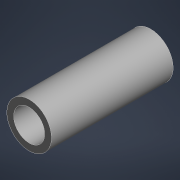
# Autodesk Inventor part: P023-Cage_arbre
Saved by Autodesk Inventor 2021.3 (Build 253353000, 353)
## iProperties
Created: 2022-06-06
Part Number: P023-Cage_arbre
Material: Générique
Document SubType Name: Modeling
Designer: Rémi Heredero
Density: 1 g/cm^3
Appearance: Par défaut
Author: Rémi Heredero
Autodesk Inventor part; units mm, degrees
ref_plane "YZ Plane" through (0, 0, 0) normal (1, 0, 0) x (0, 1, 0)
ref_plane "XZ Plane" through (0, 0, 0) normal (0, 1, 0) x (-1, 0, 0)
ref_plane "XY Plane" through (0, 0, 0) normal (0, 0, 1) x (1, 0, 0)
sketch "Sketch3" plane through (0, 0, 0) normal (1, 0, 0) x (0, 1, 0)
  line L0 (-45, 16.5) -> (-45, 11.5)
  line L1 (-45, 11.5) -> (-25, 11.5)
  line L2 (-25, 11.5) -> (-25, 11)
  line L3 (-25, 11) -> (25, 11)
  line L4 (25, 11) -> (25, 11.5)
  line L5 (25, 11.5) -> (45, 11.5)
  line L6 (45, 11.5) -> (45, 16.5)
  line L7 (45, 16.5) -> (-45, 16.5)
  line L8 (-63, 0) -> (63, 0) projected
  point P0 (0, 0)
  point P1 (0, 11)
  dimension "d0" = 5
  dimension "d1" = 20
  dimension "d2" = 50
  dimension "d6" = 23
  dimension "d7" = 22
  constraints: 16 end point, 6 perpendicular, 2 point on line, 1 collinear, 1 midpoint, 1 vertical, 1 vertical alignment
  measures "d0" distance of L5.end L6.end
  measures "d1" distance of L4.end L5.end
  measures "d2" distance of L2.end L3.end
  measures "d6" diameter of L1 L8
  measures "d7" diameter of L3 L8
revolve "Revolution1" add sketch "Sketch3" angle 360 about axis through (0, -10, 0) along (0, 1, 0)
body "Solid1"
